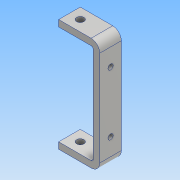
# Autodesk Inventor part: Top_End Stopper
Saved by Autodesk Inventor 2018.1 (Build 221171000, 171)
## iProperties
Created: 2019-03-22
Part Number: Top_End Stopper
Material: Aluminum 6061
Document SubType Name: Modeling
Designer: James
Density: 2.7 g/cm^3
Appearance: Aluminum - Flat
Author: James
Autodesk Inventor part; units mm, degrees
ref_plane "YZ Plane" through (0, 0, 0) normal (1, 0, 0) x (0, 1, 0)
ref_plane "XZ Plane" through (0, 0, 0) normal (0, 1, 0) x (-1, 0, 0)
ref_plane "XY Plane" through (0, 0, 0) normal (0, 0, 1) x (1, 0, 0)
sketch "Sketch1" plane through (0, 0, 0) normal (0, 1, 0) x (-1, 0, 0)
  line L0 (0, 0) -> (3, 0)
  line L1 (3, 0) -> (3, -52)
  line L2 (3, -52) -> (0, -52)
  line L3 (0, -52) -> (0, 0)
  line L4 (3, -52) -> (19, -52)
  line L5 (19, -52) -> (19, -49)
  line L6 (19, -49) -> (3, -49)
  line L7 (3, -49) -> (3, -52)
  line L8 (3, 0) -> (19, 0)
  line L9 (19, 0) -> (19, -3)
  line L10 (19, -3) -> (3, -3)
  line L11 (3, -3) -> (3, 0)
  dimension "d0" = 3
  dimension "d1" = 3
  dimension "d2" = 3
  dimension "d3" = 46
  dimension "d4" = 16
  constraints: 24 end point, 6 parallel, 3 horizontal, 3 perpendicular, 1 vertical alignment
  measures "d0" distance of L8.end L9.end
  measures "d1" distance of L4.end L5.end
  measures "d2" distance of L1.end L2.end
  measures "d3" distance between parallel lines of L6 L10
  measures "d4" distance between parallel lines of L1 L5
extrude "Extrusion1" add sketch "Sketch1" along normal blind 10
fillet "Fillet1" radius 1 2 edges at (-3, 5, -49) (-3, 5, -3)
fillet "Fillet2" radius 4 2 edges at (0, 5, -52) (0, 5, 0)
sketch "Sketch2" plane through (-19, 0, -52) normal (0, 0, -1) x (-1, 0, 0)
  line L0 (-15, 10) -> (0, 10) projected
  line L1 (0, 0) -> (0, 10) projected
  point P0 (-19, 0)
  point P1 (-5, 5)
  dimension "d9" = 5
  dimension "d10" = 5
  measures "d9" distance from line of point (-5, 5) L0
  measures "d10" distance from line of point (-5, 5) L1
hole "Hole1" at (-14, 5, -52) direction (0, 0, 1) diameter 3.4 end through all clearance for "Flat Head Machine Screw" size "M3" standard "Ansi Metric M Profile"
sketch "Sketch3" plane through (0, 0, -4) normal (1, 0, 0) x (0, 0, -1)
  line L0 (44, 10) -> (44, 0) projected
  point P0 (-4, 0)
  point P1 (8, 5)
  point P2 (36, 5)
  point P3 (44, 5)
  point P4 (45, 10)
  point P5 (-1, 10)
  dimension "d18" = 9
  dimension "d19" = 9
  constraints: 2 horizontal alignment, 1 midpoint
  measures "d18" horizontal distance of point (45, 10) point (36, 5)
  measures "d19" horizontal distance of point (-1, 10) point (8, 5)
hole "Hole2" at (0, 5, -12) at (0, 5, -40) direction (-1, 0, 0) diameter 2.4 end through all clearance for "Flat Head Machine Screw" size "M2" standard "Ansi Metric M Profile"
equation "\"d1\" = d0"
equation "\"d2\" = d0"
equation "\"d19\" = d18"
body "Solid1"
